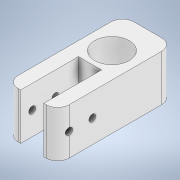
# Autodesk Inventor part: Base 1 LMU8
Saved by Autodesk Inventor 2022 (Build 260153000, 153)
## iProperties
Created: 2020-11-03
Part Number: Base 1 LMU8
Material: ABS plástico
Document SubType Name: Modeling
Designer: Mateus
Density: 1.06 g/cm^3
Appearance: Suave - Branco
Mass: 12.0952 g
Surface Area: 61.2291 cm^2
Volume: 12.8672 cm^3
Author: Mateus
## iProperties of the stored document Base 1 LMU8_3DPrint.ipt
Created: 2022-02-18
Part Number: Base 1 LMU8_3DPrint
Material: Genérico
Document SubType Name: Modeling
Designer: mathe
Density: 1 g/cm^3
Appearance: Padrão
Author: mathe
Autodesk Inventor part; units mm, degrees
ref_plane "YZ Plane" through (0, 0, 0) normal (1, 0, 0) x (0, 1, 0)
ref_plane "XZ Plane" through (0, 0, 0) normal (0, 1, 0) x (-1, 0, 0)
ref_plane "XY Plane" through (0, 0, 0) normal (0, 0, 1) x (1, 0, 0)
sketch "Esboço1" plane through (0, 0, 0) normal (0, 0, 1) x (1, 0, 0)
  line L0 (0, 0) -> (22, 0)
  line L1 (22, 0) -> (22, 20)
  line L2 (22, 20) -> (0, 20)
  line L3 (0, 20) -> (0, 0)
  dimension "d0" = 22
  dimension "d1" = 20
  constraints: 8 end point, 2 parallel, 1 horizontal, 1 perpendicular
  measures "d0" distance of L2.end L1.end
  measures "d1" distance of L1.end L0.end
extrude "Extrusão1" add sketch "Esboço1" along normal blind 50
sketch "Esboço2" plane through (0, 0, 0) normal (0, -1, 0) x (1, 0, 0)
  line L0 (0, 0) -> (0, 50) projected
  line L1 (22, 50) -> (0, 50) projected
  point P0 (11, 15.5027)
  dimension "d20" = 11
  dimension "d35" = 34.4973
  measures "d20" distance from line of L0 point (11, 15.503)
  measures "d35" distance from line of L1 point (11, 15.503)
hole "Furo1" at (11, 0, 15.5027) direction (0, 1, 0) diameter 15 end through all
fillet "Arredondamento1" radius 5 4 edges at (22, 10, 0) (0, 10, 0) (0, 10, 50) (22, 10, 50)
sketch "Esboço4" plane through (5, 20, 0) normal (0, 1, 0) x (1, 0, 0)
  line L0 (12, -50) -> (0, -50) projected
  line L1 (6, -50) -> (6, -25)
  line L2 (1, -50) -> (11, -50)
  line L3 (11, -50) -> (11, -25)
  line L4 (11, -25) -> (1, -25)
  line L5 (1, -25) -> (1, -50)
  line L6 (1, -50) -> (11, -25) construction
  line L7 (11, -50) -> (1, -25) construction
  point P0 (-5, 0)
  point P1 (6, -37.5)
  dimension "d22" = 25
  dimension "d23" = 10
  constraints: 14 end point, 4 midpoint, 2 parallel, 2 perpendicular, 1 vertical
  measures "d22" distance of L1.start L1.end
  measures "d23" distance of L2.start L2.end
extrude "Extrusão2" cut sketch "Esboço4" against normal through all
sketch "Esboço5" plane through (16, 20, 25) normal (-1, 0, 0) x (0, 0, 1)
  line L0 (25, -20) -> (25, 0) projected
  point P0 (-25, -20)
  point P1 (20, -10)
  point P2 (10, -10)
  dimension "d33" = 5
  dimension "d34" = 10
  measures "d33" distance from line of point (20, -10) L0
  measures "d34" distance of point (10, -10) point (20, -10)
hole "Furo3" at (16, 10, 45) at (16, 10, 35) direction (1, 0, 0) diameter 3 end through all both
